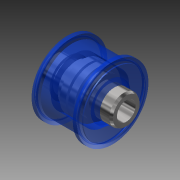
# Autodesk Inventor part: T10
Saved by Autodesk Inventor 2014 (Build 180170000, 170)
## iProperties
Created: 2014-02-02
Part Number: T10
Material: Generic
Document SubType Name: Modeling
Designer: Dream
Density: 1 g/cm^3
Appearance: Default
RuleStatus: InUse
AfterDocOpen0: CouplingSelector
Author: Dream
Autodesk Inventor part; units mm, degrees
ref_plane "YZ Plane" through (0, 0, 0) normal (1, 0, 0) x (0, 1, 0)
ref_plane "XZ Plane" through (0, 0, 0) normal (0, 1, 0) x (-1, 0, 0)
ref_plane "XY Plane" through (0, 0, 0) normal (0, 0, 1) x (1, 0, 0)
sketch "Sketch1" plane through (0, 0, 0) normal (0, 0, 1) x (1, 0, 0)
  line L0 (-69.0753, 0) -> (69.0753, 0) projected
  line L1 (0, -9.7028) -> (0, 58.2168) projected
  line L2 (0, 42.7228) -> (0, 0) construction
  line L3 (1.5875, 31.2928) -> (1.5875, 12.7)
  line L4 (1.5875, 12.7) -> (49.3395, 12.7)
  line L5 (49.3395, 12.7) -> (49.3395, 18.161)
  line L6 (18.2245, 19.812) -> (46.0375, 19.812)
  line L7 (1.5875, 31.2928) -> (9.906, 31.2928)
  line L8 (9.906, 31.2928) -> (9.906, 25.5524)
  line L9 (9.906, 25.5524) -> (18.2245, 25.5524)
  line L10 (18.2245, 25.5524) -> (18.2245, 19.812)
  line L11 (46.0375, 19.812) -> (49.3395, 18.161)
  line L12 (-1.5875, 31.2928) -> (-1.5875, 12.7)
  line L13 (-1.5875, 12.7) -> (-49.3395, 12.7)
  line L14 (-49.3395, 12.7) -> (-49.3395, 18.161)
  line L15 (-18.2245, 19.812) -> (-46.0375, 19.812)
  line L16 (-1.5875, 31.2928) -> (-9.906, 31.2928)
  line L17 (-9.906, 31.2928) -> (-9.906, 25.5524)
  line L18 (-9.906, 25.5524) -> (-18.2245, 25.5524)
  line L19 (-18.2245, 25.5524) -> (-18.2245, 19.812)
  line L20 (-46.0375, 19.812) -> (-49.3395, 18.161)
  line L21 (-33.274, 19.812) -> (-33.274, 42.5206)
  line L22 (-33.274, 42.5206) -> (-31.8389, 42.7736)
  line L23 (-31.8389, 42.7736) -> (-30.8267, 48.514)
  line L24 (-30.8267, 48.514) -> (-25.0863, 48.514)
  line L25 (-25.0863, 48.514) -> (-24.0741, 42.7736)
  line L26 (-24.0741, 42.7736) -> (0, 42.7736)
  line L27 (0, 32.8803) -> (-20.3347, 32.8803)
  line L28 (-20.3347, 32.8803) -> (-22.639, 19.812)
  circle A0 centre (-27.9565, 44.2087) radius 1.0972
  line L29 (33.274, 19.812) -> (33.274, 42.5206)
  line L30 (33.274, 42.5206) -> (31.8389, 42.7736)
  line L31 (31.8389, 42.7736) -> (30.8267, 48.514)
  line L32 (30.8267, 48.514) -> (25.0863, 48.514)
  line L33 (25.0863, 48.514) -> (24.0741, 42.7736)
  line L34 (24.0741, 42.7736) -> (0, 42.7736)
  line L35 (0, 32.8803) -> (20.3347, 32.8803)
  line L36 (20.3347, 32.8803) -> (22.639, 19.812)
  circle A1 centre (27.9565, 44.2087) radius 1.0972
  line L37 (-30.4038, 19.812) -> (-29.3916, 25.5524)
  line L38 (-29.3916, 25.5524) -> (-26.5214, 25.5524)
  line L39 (-26.5214, 25.5524) -> (-25.5092, 19.812)
  line L40 (-33.274, 19.812) -> (-30.4038, 19.812)
  line L41 (-25.5092, 19.812) -> (-22.639, 19.812)
  line L42 (30.4038, 19.812) -> (29.3916, 25.5524)
  line L43 (29.3916, 25.5524) -> (26.5214, 25.5524)
  line L44 (26.5214, 25.5524) -> (25.5092, 19.812)
  line L45 (33.274, 19.812) -> (30.4038, 19.812)
  line L46 (25.5092, 19.812) -> (22.639, 19.812)
  line L47 (-27.9565, 48.514) -> (-27.9565, 42.7736) construction
  dimension "d0" = 1.5875
  dimension "ShaftRadii" = 12.7
  dimension "d2" = 47.752
  dimension "d3" = 19.812
  dimension "d4" = 48.514
  dimension "d5" = 33.274
  dimension "d9" = 1.651
  dimension "d10" = 3.302
  dimension "d11" = 28.702
  dimension "d12" = 1.5875
  dimension "d13" = 5.7404
  dimension "d14" = 5.7404
  dimension "d15" = 5.7404
  dimension "d17" = 80
  dimension "d19" = 80
  dimension "d20" = 80
  dimension "d21" = 1.4351
  dimension "d22" = 4.3053
  dimension "d23" = 2.1945
  dimension "d24" = 5.7404
  dimension "d25" = 80
  dimension "d26" = 80
  dimension "d27" = 5.7404
  dimension "d28" = 80
  dimension "d30" = 2.8702
  dimension "d31" = 2.8702
  dimension "d32" = 2.8702
  dimension "d33" = 8.3185
  dimension "d34" = 8.3185
  constraints: 92 end point, 22 symmetric about line, 9 point on line, 8 parallel, 6 perpendicular, 3 collinear, 2 centre point, 1 midpoint, 1 other
  measures "d0" distance between parallel lines of L1 L3
  measures "ShaftRadii" distance between parallel lines of L0 L4
  measures "d2" distance of L3.end L4.end
  measures "d3" distance between parallel lines of L0 L6
  measures "d4" distance between parallel lines of L0 L24
  measures "d5" distance between parallel lines of L2 L21
  measures "d9" vertical distance of L6.end L5.end
  measures "d10" horizontal distance of L6.end L5.end
  measures "d11" distance between parallel lines of L15 L24
  measures "d12" distance between parallel lines of L27 L16
  measures "d13" distance between parallel lines of L26 L24
  measures "d14" distance of L18.end L15.start
  measures "d15" distance of L16.end L17.end
  measures "d17" angle of L25 L24
  measures "d19" angle of L24 L23
  measures "d20" angle of L22 L21
  measures "d21" horizontal distance of L21.end L22.end
  measures "d22" distance from line of L24 A0.centre
  measures "d23" diameter of A0
  measures "d24" distance of L23.end L24.end
  measures "d25" angle of L15 L37
  measures "d26" angle of L15 L39
  measures "d27" distance between parallel lines of L15 L38
  measures "d28" angle of L15 L28
  measures "d30" distance of L37.end L38.end
  measures "d31" distance of L21.start L37.start
  measures "d32" distance of L39.end L28.end
  measures "d33" distance of L17.end L18.end
  measures "d34" distance of L12.start L16.end
revolve "Revolution1 - Hub" add sketch "Sketch1" angle 360 about axis through (-10, 0, 0) along (1, 0, 0) contours L15 L19 L18 L17 L16 L12 L13 L14 L20 | L6 L11 L5 L4 L3 L7 L8 L9 L10
revolve "Revolution3" add sketch "Sketch1" angle 360 about axis through (-10, 0, 0) along (1, 0, 0) separate body contours L27 L28 L15 L39 L38 L37 L21 L22 L23 L24 L25 L26 L1 | L1 L34 L33 L32 L31 L30 L29 L6 L42 L43 L44 L36 L35
equation "\"d0\" = 0.5 * Gap"
equation "\"ShaftRadii\" = 0.5 * ShaftDia"
equation "\"d2\" = d_C"
equation "\"d3\" = 0.5 * d_D"
equation "\"d4\" = 0.5 * d_A"
equation "\"d5\" = 0.5 * d_J"
equation "\"d9\" = 0.0833333 * d3"
equation "\"d10\" = 2 * d9"
equation "\"d12\" = 0.5 * Gap"
equation "\"d13\" = 0.2 * d11"
equation "\"d14\" = 0.2 * d11"
equation "\"d15\" = 0.2 * d11"
equation "\"d19\" = d17"
equation "\"d20\" = d17"
equation "\"d21\" = 0.25 * d13"
equation "\"d22\" = 0.75 * d13"
equation "\"d24\" = d13"
equation "\"d25\" = d17"
equation "\"d26\" = d17"
equation "\"d27\" = d14"
equation "\"d28\" = d17"
equation "\"d30\" = 0.5 * d24"
equation "\"d31\" = d30"
equation "\"d32\" = d30"
equation "\"d33\" = 0.25 * d5"
equation "\"d34\" = 0.25 * d5"
equation "\"Gap\" = 3.175"
equation "\"d_A\" = 97.028"
equation "\"d_B\" = 98.552"
equation "\"d_C\" = 47.752"
equation "\"d_D\" = 39.624"
equation "\"d_J\" = 66.548"
equation "\"d_S\" = 39.116"
equation "\"d_F\" = 0"
equation "\"ShaftDia\" = 25.4"
